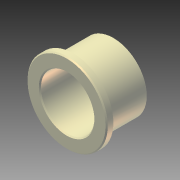
# Autodesk Inventor part: Chassis_Washer_AndyMark_am-0947
Saved by Autodesk Inventor 2012 (Build 160160000, 160)
## iProperties
Category: Drive Base Kit
Company: Autodesk Inc.
Created: 2011-12-28
Part Number: Chassis_Washer_AndyMark_am-0947
Material: Nylon-6/6
Document SubType Name: Modeling
Designer: Autodesk Inc.
Density: 1.13 g/cm^3
Catalog Web Link: www.andymark.com
Description: Shoulder Washer, 1/2" ID
Vendor: AndyMark
Mass: 1.04589 g
Surface Area: 13.0941 cm^2
Volume: 0.925564 cm^3
Author: Autodesk Inc.
Autodesk Inventor part; units mm, degrees
ref_plane "YZ Plane" through (0, 0, 0) normal (1, 0, 0) x (0, 1, 0)
ref_plane "XZ Plane" through (0, 0, 0) normal (0, 1, 0) x (-1, 0, 0)
ref_plane "XY Plane" through (0, 0, 0) normal (0, 0, 1) x (1, 0, 0)
sketch "Sketch1" plane through (0, 0, 0) normal (0, 0, 1) x (1, 0, 0)
  circle A0 centre (0, 0) radius 6.35
  circle A1 centre (0, 0) radius 7.9375
  circle A2 centre (0, 0) radius 9.525
  dimension "d0" = 12.7
  dimension "d1" = 15.875
  dimension "d2" = 19.05
  constraints: 3 centre point, 3 coincident
  measures "d0" diameter of A0
  measures "d1" diameter of A1
  measures "d2" diameter of A2
extrude "Extrusion1" add sketch "Sketch1" against normal blind 9.525 contours A1
extrude "Extrusion2" add sketch "Sketch1" along normal blind 1.5875 contours A1 | A2
chamfer "Chamfer1" distance 0.254 angle 45 3 edges at (-9.525, 0, 1.5875) (-6.35, 0, 1.5875) (-6.35, 0, -9.525)
body "Solid1"
